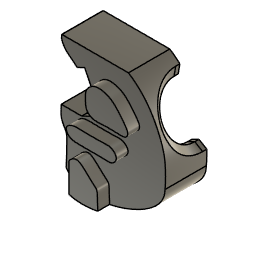
O4 Lite Cam Crux35 25° (Autodesk Fusion 360 design; units mm, degrees)
Autodesk Fusion 360 part; units mm, degrees
sketch "Skizze1" plane through (0, 0, 0) normal (0, 1, 0) x (1, 0, 0)
  spline S0 degree 5 poles (-4.5243, -6.4632) (-4.5158, -6.5005) (-4.4961, -6.5754) (-4.4576, -6.6893) (-4.387, -6.8464) (-4.2661, -7.0503) (-4.1148, -7.2567) (-3.9364, -7.4581) (-3.7332, -7.6461) (-3.5066, -7.8125) (-3.2573, -7.9501) (-2.9862, -8.0532) (-2.6953, -8.1181) (-2.3883, -8.144) (-2.0711, -8.1333) (-1.7509, -8.0908) (-1.4354, -8.0221) (-1.1309, -7.9326) (-0.8422, -7.8263) (-0.5706, -7.7044) (-0.3132, -7.5642) (-0.0646, -7.4007) (0.1819, -7.2085) (0.4324, -6.983) (0.6912, -6.7225) (0.9588, -6.4299) (1.2309, -6.1139) (1.4992, -5.7875) (1.7538, -5.4654) (1.9842, -5.1623) (2.1811, -4.8902) (2.3382, -4.6566) (2.4535, -4.4623) (2.5313, -4.2987) (2.5788, -4.1529) (2.6034, -4.0118) (2.6095, -3.8666) (2.5953, -3.7172) (2.5566, -3.5686) (2.4882, -3.4288) (2.3871, -3.3059) (2.253, -3.2064) (2.0873, -3.1347) (1.8932, -3.091) (1.6755, -3.0713) (1.4391, -3.0687) (1.1878, -3.0758) (0.9237, -3.0858) (0.6453, -3.0951) (0.3485, -3.1029) (0.0288, -3.1095) (-0.3168, -3.1156) (-0.6877, -3.1201) (-1.0785, -3.1204) (-1.4748, -3.1083) (-1.8652, -3.0861) (-2.2403, -3.0621) (-2.5925, -3.048) (-2.9161, -3.0556) (-3.2074, -3.0942) (-3.4642, -3.1674) (-3.6861, -3.2699) (-3.8741, -3.3904) (-4.0304, -3.5174) (-4.1583, -3.6426) (-4.2619, -3.7671) (-4.3457, -3.9025) (-4.4138, -4.0635) (-4.4694, -4.2624) (-4.5133, -4.5016) (-4.5449, -4.7733) (-4.5636, -5.0635) (-4.5705, -5.3549) (-4.5688, -5.6301) (-4.5684, -5.8739) (-4.5678, -6.0868) (-4.5607, -6.2401) (-4.5469, -6.3516) (-4.5327, -6.4259) (-4.5243, -6.4632) knots 0 0 0 0 0 0 0.01333333 0.02666667 0.04 0.05333333 0.06666667 0.08 0.09333333 0.10666667 0.12 0.13333333 0.14666667 0.16 0.17333333 0.18666667 0.2 0.21333333 0.22666667 0.24 0.25333333 0.26666667 0.28 0.29333333 0.30666667 0.32 0.33333333 0.34666667 0.36 0.37333333 0.38666667 0.4 0.41333333 0.42666667 0.44 0.45333333 0.46666667 0.48 0.49333333 0.50666667 0.52 0.53333333 0.54666667 0.56 0.57333333 0.58666667 0.6 0.61333333 0.62666667 0.64 0.65333333 0.66666667 0.68 0.69333333 0.70666667 0.72 0.73333333 0.74666667 0.76 0.77333333 0.78666667 0.8 0.81333333 0.82666667 0.84 0.85333333 0.86666667 0.88 0.89333333 0.90666667 0.92 0.93333333 0.94666667 0.96 0.97333333 0.98666667 1 1 1 1 1 1
  line L0 (-4.5692, -4.1589) -> (-4.5692, -6.8679)
  line L1 (0.5002, -3.1248) -> (-2.2874, -3.1136)
  spline S1 degree 5 poles (-7.828, 0.5821) (-7.8299, 0.5449) (-7.8288, 0.4718) (-7.8125, 0.3664) (-7.7619, 0.2361) (-7.6561, 0.0903) (-7.5159, -0.0401) (-7.3514, -0.156) (-7.1728, -0.2565) (-6.9877, -0.34) (-6.7987, -0.4054) (-6.6005, -0.4522) (-6.3797, -0.4819) (-6.1198, -0.4966) (-5.8052, -0.4996) (-5.4254, -0.4942) (-4.9796, -0.4843) (-4.4781, -0.4732) (-3.9383, -0.4641) (-3.3823, -0.4595) (-2.8342, -0.4609) (-2.3169, -0.4687) (-1.8502, -0.4819) (-1.4472, -0.4977) (-1.1118, -0.5117) (-0.8364, -0.517) (-0.6063, -0.5061) (-0.4046, -0.472) (-0.2155, -0.4094) (-0.03, -0.3161) (0.1518, -0.1938) (0.3238, -0.0463) (0.4756, 0.1215) (0.5947, 0.3046) (0.6695, 0.4998) (0.6907, 0.7037) (0.6542, 0.9119) (0.5635, 1.1178) (0.4316, 1.3115) (0.2757, 1.4821) (0.1115, 1.6204) (-0.0521, 1.7209) (-0.2189, 1.7847) (-0.4024, 1.8178) (-0.6194, 1.8292) (-0.8847, 1.8276) (-1.2051, 1.8201) (-1.5798, 1.811) (-2.0028, 1.8031) (-2.4635, 1.7979) (-2.9489, 1.7955) (-3.4452, 1.7953) (-3.9385, 1.7965) (-4.4173, 1.7979) (-4.8728, 1.7984) (-5.2979, 1.7967) (-5.6883, 1.7909) (-6.0413, 1.7786) (-6.3565, 1.7565) (-6.6355, 1.7204) (-6.8815, 1.6647) (-7.0991, 1.5836) (-7.2923, 1.4727) (-7.463, 1.3304) (-7.6098, 1.1597) (-7.7268, 0.9697) (-7.7902, 0.8116) (-7.8175, 0.695) (-7.8261, 0.6193) (-7.828, 0.5821) knots 0 0 0 0 0 0 0.01538462 0.03076923 0.04615385 0.06153846 0.07692308 0.09230769 0.10769231 0.12307692 0.13846154 0.15384615 0.16923077 0.18461538 0.2 0.21538462 0.23076923 0.24615385 0.26153846 0.27692308 0.29230769 0.30769231 0.32307692 0.33846154 0.35384615 0.36923077 0.38461538 0.4 0.41538462 0.43076923 0.44615385 0.46153846 0.47692308 0.49230769 0.50769231 0.52307692 0.53846154 0.55384615 0.56923077 0.58461538 0.6 0.61538462 0.63076923 0.64615385 0.66153846 0.67692308 0.69230769 0.70769231 0.72307692 0.73846154 0.75384615 0.76923077 0.78461538 0.8 0.81538462 0.83076923 0.84615385 0.86153846 0.87692308 0.89230769 0.90769231 0.92307692 0.93846154 0.95384615 0.96923077 0.98461538 1 1 1 1 1 1
  spline S2 degree 5 poles (0.7271, -10.9082) (0.7967, -10.8654) (0.9365, -10.7771) (1.1485, -10.6366) (1.4356, -10.4329) (1.8018, -10.1509) (2.1746, -9.8407) (2.553, -9.5012) (2.9346, -9.1301) (3.3165, -8.7247) (3.6952, -8.2828) (4.0668, -7.8031) (4.4273, -7.2869) (4.7731, -6.7381) (5.1012, -6.1651) (5.4088, -5.5784) (5.6938, -4.9891) (5.9542, -4.4067) (6.1884, -3.8372) (6.3948, -3.2812) (6.5719, -2.7314) (6.7184, -2.1753) (6.8338, -1.5992) (6.9185, -0.9921) (6.9744, -0.3496) (7.005, 0.3223) (7.0162, 1.0029) (7.0134, 1.663) (6.9995, 2.2713) (6.972, 2.8004) (6.9209, 3.2327) (6.8257, 3.5676) (6.6546, 3.8249) (6.3782, 4.033) (5.9781, 4.2204) (5.4612, 4.4038) (4.8576, 4.5875) (4.2094, 4.7688) (3.5631, 4.9413) (2.9601, 5.0993) (2.4284, 5.2416) (1.9725, 5.3758) (1.5805, 5.5149) (1.235, 5.6722) (0.9208, 5.8567) (0.6377, 6.0672) (0.4005, 6.2933) (0.2263, 6.5254) (0.1239, 6.7635) (0.0824, 7.0258) (0.0801, 7.3402) (0.0932, 7.7348) (0.1056, 8.2279) (0.1096, 8.8275) (0.1027, 9.5351) (0.0866, 10.3475) (0.0692, 11.0771) (0.0552, 11.6666) (0.0458, 12.0782) (0.041, 12.2887) knots 0 0 0 0 0 0 0.018182 0.036364 0.054545 0.072727 0.090909 0.109091 0.127273 0.145455 0.163636 0.181818 0.2 0.218182 0.236364 0.254545 0.272727 0.290909 0.309091 0.327273 0.345455 0.363636 0.381818 0.4 0.418182 0.436364 0.454545 0.472727 0.490909 0.509091 0.527273 0.545455 0.563636 0.581818 0.6 0.618182 0.636364 0.654545 0.672727 0.690909 0.709091 0.727273 0.745455 0.763636 0.781818 0.8 0.818182 0.836364 0.854545 0.872727 0.890909 0.909091 0.927273 0.945455 0.963636 0.981818 1 1 1 1 1 1
  line L2 (0.1295, 8.393) -> (-0.0476, 16.1843)
  spline S3 degree 5 poles (-10.5835, -10.8639) (-10.593, -10.8262) (-10.6087, -10.7498) (-10.6228, -10.632) (-10.6224, -10.4684) (-10.5903, -10.2535) (-10.5273, -10.0295) (-10.4348, -9.7988) (-10.3155, -9.5657) (-10.1726, -9.3361) (-10.0106, -9.1161) (-9.8339, -8.911) (-9.6472, -8.7244) (-9.4548, -8.5569) (-9.2607, -8.4053) (-9.0679, -8.2637) (-8.8786, -8.1254) (-8.6936, -7.9843) (-8.5125, -7.8363) (-8.3328, -7.6812) (-8.1517, -7.5217) (-7.9666, -7.3618) (-7.7768, -7.2058) (-7.5843, -7.057) (-7.3954, -6.9161) (-7.219, -6.7819) (-7.0644, -6.6516) (-6.9396, -6.5213) (-6.849, -6.3866) (-6.7922, -6.2435) (-6.7666, -6.0893) (-6.77, -5.9243) (-6.8027, -5.7531) (-6.8675, -5.5835) (-6.9667, -5.4229) (-7.1011, -5.2762) (-7.2676, -5.1432) (-7.4601, -5.0192) (-7.6714, -4.898) (-7.894, -4.7732) (-8.1219, -4.6398) (-8.3515, -4.4965) (-8.5808, -4.3444) (-8.8086, -4.1861) (-9.0343, -4.0251) (-9.2567, -3.865) (-9.4735, -3.7085) (-9.6808, -3.5567) (-9.8746, -3.4095) (-10.0503, -3.2646) (-10.2043, -3.1176) (-10.334, -2.9615) (-10.4384, -2.7872) (-10.518, -2.5853) (-10.5747, -2.3487) (-10.6116, -2.0738) (-10.6333, -1.7633) (-10.6449, -1.4252) (-10.6516, -1.0708) (-10.6581, -0.7128) (-10.6673, -0.3634) (-10.6804, -0.0325) (-10.6954, 0.2745) (-10.707, 0.5582) (-10.7075, 0.8239) (-10.6888, 1.0793) (-10.6445, 1.3319) (-10.5707, 1.5875) (-10.4688, 1.8472) (-10.3459, 2.1064) (-10.2126, 2.358) (-10.0811, 2.5943) (-9.9627, 2.8103) (-9.8663, 3.0054) (-9.7953, 3.1868) (-9.7489, 3.368) (-9.7229, 3.5636) (-9.7118, 3.7862) (-9.7104, 4.0413) (-9.7147, 4.3254) (-9.7214, 4.6299) (-9.7286, 4.9432) (-9.7349, 5.2537) (-9.7398, 5.5523) (-9.7434, 5.8358) (-9.7467, 6.1077) (-9.7506, 6.3758) (-9.7564, 6.65) (-9.7651, 6.9404) (-9.7773, 7.2548) (-9.7929, 7.5966) (-9.8113, 7.9641) (-9.8311, 8.3522) (-9.851, 8.7527) (-9.8693, 9.1564) (-9.8847, 9.5536) (-9.8961, 9.9353) (-9.9029, 10.2945) (-9.9054, 10.6272) (-9.9048, 10.9321) (-9.9035, 11.2096) (-9.9056, 11.4609) (-9.9168, 11.687) (-9.9451, 11.8882) (-10.0009, 12.0625) (-10.0906, 12.2077) (-10.2072, 12.3219) (-10.3222, 12.4063) (-10.3783, 12.4655) (-10.3182, 12.5059) (-10.1184, 12.5327) (-9.7918, 12.5498) (-9.3741, 12.5607) (-8.9151, 12.5693) (-8.4684, 12.5807) (-8.081, 12.6023) (-7.7844, 12.6437) (-7.5819, 12.7189) (-7.4552, 12.8428) (-7.3767, 13.0267) (-7.319, 13.2753) (-7.2672, 13.5814) (-7.2235, 13.9252) (-7.1974, 14.2804) (-7.1996, 14.6186) (-7.2347, 14.914) (-7.2939, 15.1483) (-7.3479, 15.3154) (-7.3413, 15.426) (-7.2152, 15.4984) (-6.9287, 15.5508) (-6.4787, 15.5938) (-5.8906, 15.6324) (-5.2103, 15.6666) (-4.4962, 15.6937) (-3.8111, 15.709) (-3.2139, 15.7075) (-2.7517, 15.6852) (-2.4513, 15.6403) (-2.312, 15.575) (-2.295, 15.4968) (-2.3237, 15.4181) (-2.3343, 15.3408) (-2.3181, 15.2438) (-2.295, 15.0995) (-2.2824, 14.8939) (-2.2806, 14.6331) (-2.2816, 14.3355) (-2.2708, 14.0265) (-2.2326, 13.7321) (-2.1539, 13.4735) (-2.0281, 13.2609) (-1.8548, 13.0959) (-1.6384, 12.9743) (-1.3877, 12.8884) (-1.1145, 12.8294) (-0.8332, 12.7902) (-0.5592, 12.7652) (-0.3075, 12.7499) (-0.0915, 12.7414) (0.0784, 12.7374) (0.1729, 12.7371) (0.2198, 12.7383) (0.2404, 12.7398) (0.248, 12.7407) knots 0 0 0 0 0 0 0.00625 0.0125 0.01875 0.025 0.03125 0.0375 0.04375 0.05 0.05625 0.0625 0.06875 0.075 0.08125 0.0875 0.09375 0.1 0.10625 0.1125 0.11875 0.125 0.13125 0.1375 0.14375 0.15 0.15625 0.1625 0.16875 0.175 0.18125 0.1875 0.19375 0.2 0.20625 0.2125 0.21875 0.225 0.23125 0.2375 0.24375 0.25 0.25625 0.2625 0.26875 0.275 0.28125 0.2875 0.29375 0.3 0.30625 0.3125 0.31875 0.325 0.33125 0.3375 0.34375 0.35 0.35625 0.3625 0.36875 0.375 0.38125 0.3875 0.39375 0.4 0.40625 0.4125 0.41875 0.425 0.43125 0.4375 0.44375 0.45 0.45625 0.4625 0.46875 0.475 0.48125 0.4875 0.49375 0.5 0.50625 0.5125 0.51875 0.525 0.53125 0.5375 0.54375 0.55 0.55625 0.5625 0.56875 0.575 0.58125 0.5875 0.59375 0.6 0.60625 0.6125 0.61875 0.625 0.63125 0.6375 0.64375 0.65 0.65625 0.6625 0.66875 0.675 0.68125 0.6875 0.69375 0.7 0.70625 0.7125 0.71875 0.725 0.73125 0.7375 0.74375 0.75 0.75625 0.7625 0.76875 0.775 0.78125 0.7875 0.79375 0.8 0.80625 0.8125 0.81875 0.825 0.83125 0.8375 0.84375 0.85 0.85625 0.8625 0.86875 0.875 0.88125 0.8875 0.89375 0.9 0.90625 0.9125 0.91875 0.925 0.93125 0.9375 0.94375 0.95 0.95625 0.9625 0.96875 0.975 0.98125 0.9875 0.99375 1 1 1 1 1 1
  spline S4 degree 5 poles (-10.5835, -10.8639) (-10.58, -10.8789) (-10.5697, -10.9076) (-10.5442, -10.9472) (-10.4901, -10.9926) (-10.3892, -11.0376) (-10.2564, -11.0718) (-10.0953, -11.0974) (-9.9126, -11.1185) (-9.7173, -11.1407) (-9.5195, -11.17) (-9.3291, -11.212) (-9.1547, -11.2716) (-9.0019, -11.3517) (-8.8735, -11.4531) (-8.7699, -11.5755) (-8.6903, -11.7173) (-8.6331, -11.877) (-8.5967, -12.053) (-8.5799, -12.244) (-8.5817, -12.4493) (-8.5976, -12.6245) (-8.6174, -12.762) (-8.6341, -12.8563) (-8.6433, -12.9041) knots 0 0 0 0 0 0 0.05 0.1 0.15 0.2 0.25 0.3 0.35 0.4 0.45 0.5 0.55 0.6 0.65 0.7 0.75 0.8 0.85 0.9 0.95 1 1 1 1 1 1
  line L3 (-8.6433, -12.9041) -> (1.0723, -12.9041)
  line L4 (0.7271, -10.9082) -> (0.7271, -12.9041)
  line L5 (0.041, 12.2887) -> (0.0307, 12.7389)
  spline S5 degree 5 poles (-7.3471, 5.0204) (-7.3368, 5.0013) (-7.3139, 4.9624) (-7.2723, 4.9023) (-7.2022, 4.819) (-7.0909, 4.7099) (-6.9574, 4.5983) (-6.8045, 4.4885) (-6.637, 4.388) (-6.4609, 4.3055) (-6.282, 4.249) (-6.1051, 4.2247) (-5.9336, 4.2347) (-5.768, 4.2765) (-5.6073, 4.3456) (-5.4491, 4.4366) (-5.29, 4.5454) (-5.1262, 4.6706) (-4.9538, 4.8134) (-4.7697, 4.9751) (-4.5719, 5.1566) (-4.3602, 5.3568) (-4.137, 5.5713) (-3.9072, 5.7915) (-3.6777, 6.0072) (-3.4561, 6.2083) (-3.25, 6.3867) (-3.0664, 6.5386) (-2.9105, 6.6658) (-2.7847, 6.7787) (-2.6891, 6.8941) (-2.6212, 7.0302) (-2.5773, 7.2024) (-2.5523, 7.418) (-2.5403, 7.674) (-2.5355, 7.9606) (-2.5327, 8.2638) (-2.5275, 8.5679) (-2.5177, 8.8589) (-2.503, 9.1266) (-2.4863, 9.3678) (-2.4724, 9.5842) (-2.467, 9.7804) (-2.4758, 9.9615) (-2.5031, 10.1314) (-2.5511, 10.2904) (-2.62, 10.4356) (-2.709, 10.5628) (-2.8174, 10.6681) (-2.9453, 10.7498) (-3.0942, 10.8089) (-3.2659, 10.8481) (-3.4616, 10.8716) (-3.6814, 10.8837) (-3.9234, 10.8886) (-4.1844, 10.8905) (-4.46, 10.8924) (-4.7449, 10.8966) (-5.0331, 10.904) (-5.3186, 10.9142) (-5.5952, 10.9248) (-5.8572, 10.932) (-6.0998, 10.9319) (-6.3192, 10.9202) (-6.5131, 10.8935) (-6.6812, 10.8495) (-6.8254, 10.7879) (-6.9487, 10.7091) (-7.0547, 10.6145) (-7.1464, 10.5053) (-7.2256, 10.3823) (-7.2798, 10.2731) (-7.3154, 10.1853) (-7.3369, 10.124) (-7.3471, 10.0927) knots 0 0 0 0 0 0 0.01428571 0.02857143 0.04285714 0.05714286 0.07142857 0.08571429 0.1 0.11428571 0.12857143 0.14285714 0.15714286 0.17142857 0.18571429 0.2 0.21428571 0.22857143 0.24285714 0.25714286 0.27142857 0.28571429 0.3 0.31428571 0.32857143 0.34285714 0.35714286 0.37142857 0.38571429 0.4 0.41428571 0.42857143 0.44285714 0.45714286 0.47142857 0.48571429 0.5 0.51428571 0.52857143 0.54285714 0.55714286 0.57142857 0.58571429 0.6 0.61428571 0.62857143 0.64285714 0.65714286 0.67142857 0.68571429 0.7 0.71428571 0.72857143 0.74285714 0.75714286 0.77142857 0.78571429 0.8 0.81428571 0.82857143 0.84285714 0.85714286 0.87142857 0.88571429 0.9 0.91428571 0.92857143 0.94285714 0.95714286 0.97142857 0.98571429 1 1 1 1 1 1
  line L6 (-7.3471, 5.0204) -> (-7.3471, 10.0927)
  line L7 (0.7271, -10.9082) -> (-10.5662, -10.9082)
  spline S6 degree 5 poles (1.0592, 5.7812) (0.6047, 5.9716) (-0.3091, 6.3124) (-1.6948, 6.7027) (-3.5583, 6.9827) (-5.8366, 6.8357) (-7.5331, 6.1361) (-8.682, 5.1382) (-9.3829, 4.2305) (-9.717, 3.7159) knots 0 0 0 0 0 0 0.2 0.4 0.6 0.8 1 1 1 1 1 1
  line L8 (2.1287, 5.3329) -> (-0.0104, 6.2295)
  line L9 (-8.9784, 4.8533) -> (-10.4557, 2.5786)
  spline S7 degree 5 poles (6.9248, 3.125) (6.9282, 3.4844) (6.8431, 4.1897) (6.4398, 5.2074) (5.3882, 6.4762) (3.4261, 7.8713) (1.0807, 9.0146) (-1.3779, 9.8419) (-3.7125, 10.2975) (-5.773, 10.3603) (-7.4988, 10.0428) (-8.5998, 9.5018) (-9.2721, 8.9435) (-9.6531, 8.5047) (-9.8268, 8.2686) knots 0 0 0 0 0 0 0.1 0.2 0.3 0.4 0.5 0.6 0.7 0.8 0.9 1 1 1 1 1 1
  line L10 (6.911, 1.683) -> (6.9386, 4.5671)
  point P0 (-4.0016, -7.3793)
  point P1 (-2.6808, -8.1099)
  point P2 (-0.8486, -7.8233)
  point P3 (0.7025, -6.7049)
  point P4 (2.3324, -4.6591)
  point P5 (2.5965, -4.0297)
  point P6 (2.5347, -3.5351)
  point P7 (2.1132, -3.1529)
  point P8 (1.0847, -3.0799)
  point P9 (-0.8936, -3.1192)
  point P10 (-3.2485, -3.1136)
  point P11 (-4.114, -3.6025)
  point P12 (-4.4343, -4.1477)
  point P13 (-4.5692, -5.5134)
  point P14 (-7.563, 0.0092)
  point P15 (-6.8669, -0.379)
  point P16 (-5.6039, -0.496)
  point P17 (-1.4945, -0.496)
  point P18 (-0.2685, -0.4221)
  point P19 (0.4585, 0.1139)
  point P20 (0.6434, 0.9025)
  point P21 (0.0766, 1.6356)
  point P22 (-0.6689, 1.8266)
  point P23 (-3.5954, 1.7958)
  point P24 (-6.4602, 1.7404)
  point P25 (-7.4398, 1.3399)
  point P26 (2.3872, -9.6465)
  point P27 (4.4678, -7.2117)
  point P28 (6.2386, -3.6923)
  point P29 (6.969, -0.3279)
  point P30 (6.9248, 3.125)
  point P31 (6.2165, 4.099)
  point P32 (2.8963, 5.1171)
  point P33 (1.0592, 5.7812)
  point P34 (0.2402, 6.5337)
  point P35 (0.0852, 7.4412)
  point P36 (-10.4741, -9.9052)
  point P37 (-9.6406, -8.7243)
  point P38 (-8.6751, -7.9672)
  point P39 (-7.7444, -7.1823)
  point P40 (-6.9734, -6.5502)
  point P41 (-6.7719, -6.0432)
  point P42 (-6.9873, -5.4111)
  point P43 (-7.8694, -4.786)
  point P44 (-9.1544, -3.9385)
  point P45 (-10.1546, -3.1606)
  point P46 (-10.5835, -2.2576)
  point P47 (-10.6825, -0.0002)
  point P48 (-10.5835, 1.528)
  point P49 (-9.9324, 2.8755)
  point P50 (-9.717, 3.7159)
  point P51 (-9.7379, 5.4455)
  point P52 (-9.7719, 7.1063)
  point P53 (-9.8968, 10.0068)
  point P54 (-9.9245, 11.7137)
  point P55 (-10.2021, 12.3105)
  point P56 (-10.3409, 12.477)
  point P57 (-8.0233, 12.6158)
  point P58 (-7.3432, 13.1848)
  point P59 (-7.2877, 15.1138)
  point P60 (-7.1906, 15.4885)
  point P61 (-2.3611, 15.5857)
  point P62 (-2.3194, 15.4191)
  point P63 (-2.3056, 15.1555)
  point P64 (-2.2223, 13.7399)
  point P65 (-1.3758, 12.8934)
  point P66 (-0.0435, 12.7407)
  point P67 (-10.2162, -11.0761)
  point P68 (-9.2385, -11.2462)
  point P69 (-8.6646, -11.7988)
  point P70 (-6.9606, 4.605)
  point P71 (-6.1684, 4.2379)
  point P72 (-5.4341, 4.4504)
  point P73 (-4.41, 5.3103)
  point P74 (-3.0091, 6.5856)
  point P75 (-2.5936, 7.1556)
  point P76 (-2.5164, 8.8561)
  point P77 (-2.4874, 10.0154)
  point P78 (-2.7676, 10.6144)
  point P79 (-3.4342, 10.8656)
  point P80 (-5.0187, 10.9043)
  point P81 (-6.4776, 10.8946)
  point P82 (-7.0476, 10.6144)
  point P83 (-2.4874, 10.0154)
  constraint midpoint P13 L0
  constraint midpoint P9 L1
  constraint midpoint S2.end L2
  constraint horizontal L3
  constraint coincident L3 L4.end
  constraint perpendicular L3 L4
  constraint coincident S3 L5.end
  constraint vertical L6
  constraint horizontal L7
  constraint coincident S4 L7.end
  constraint coincident P33 S6.start
  constraint coincident P50 S6.end
  constraint midpoint P33 L8
  constraint coincident S2 L8.start
  constraint midpoint P50 L9
  constraint coincident P30 S7.start
  constraint coincident P83 P77
  constraint midpoint P30 L10
  constraint coincident S3 S7.end
extrude "Extrusion1" add sketch "Skizze1" along normal blind 1 contours S0 | S1 | S2 S3 S4 S5 L6 L7 S6 | S2 L2 S7 | S4 L3 L4 L7 | S2 S5 S6 S7 | S2 L2 S3 L5 S5 L6 S7 | S3 L6 S6 S7 | S5 L6 S6 S7 | S5 L6 S6 | S5 L6 S7 makes body 1
extrude "Extrusion2" add sketch "Skizze1" along normal blind 3 contours S0 | S1 | S5 L6 S6 S7 | S5 L6 S6 | S5 L6 S7 bodies 1
delete_body "Körper entfernen1" bodies 1
sketch "Skizze2" plane through (0, 0, 0) normal (1, 0, 0) x (0, 1, 0)
  line L0 (0, 0) -> (14, 0)
  circle A0 centre (7, 0) radius 4.3
  line L1 (12.5, -5.5) -> (1.5, -5.5)
  line L2 (1.5, -5.5) -> (1.5, 5.5)
  line L3 (1.5, 5.5) -> (12.5, 5.5)
  line L4 (12.5, 5.5) -> (12.5, -5.5)
  line L5 (12.5, -5.5) -> (1.5, 5.5) construction
  line L6 (1.5, -5.5) -> (12.5, 5.5) construction
  line L7 (13.1, -6.1) -> (0.9, -6.1)
  line L8 (0.9, -6.1) -> (0.9, 6.1)
  line L9 (0.9, 6.1) -> (13.1, 6.1)
  line L10 (13.1, 6.1) -> (13.1, -6.1)
  line L11 (13.1, -6.1) -> (0.9, 6.1) construction
  line L12 (0.9, -6.1) -> (13.1, 6.1) construction
  line L13 (13.25, -8.25) -> (0.75, -8.25)
  line L14 (0.75, -8.25) -> (0.75, 8.25)
  line L15 (0.75, 8.25) -> (13.25, 8.25)
  line L16 (13.25, 8.25) -> (13.25, -8.25)
  line L17 (13.25, -8.25) -> (0.75, 8.25) construction
  line L18 (0.75, -8.25) -> (13.25, 8.25) construction
  point P0 (7, 0)
  point P1 (7, 0)
  point P2 (7, 0)
  dimension "d5" = 14
  dimension "d6" = 8.6
  dimension "d7" = 11
  dimension "d8" = 11
  dimension "d9" = 12.2
  dimension "d10" = 12.2
  dimension "d11" = 12.5
  dimension "d12" = 16.5
  constraint coincident L0.start origin
  constraint horizontal L0
  constraint midpoint L0 P2
  constraint horizontal L1
  constraint perpendicular L1 L2
  constraint parallel L1 L3
  constraint parallel L2 L4
  constraint coincident L5 P2
  constraint coincident L6 P2
  constraint coincident P2 P1
  constraint horizontal L7
  constraint perpendicular L7 L8
  constraint parallel L7 L9
  constraint parallel L8 L10
  constraint coincident L11 P2
  constraint coincident L12 P2
  constraint horizontal L13
  constraint perpendicular L13 L14
  constraint parallel L13 L15
  constraint parallel L14 L16
  constraint coincident L17 P2
  constraint coincident L18 P2
  measures "d5" distance of L0.start L0.end
  measures "d6" diameter of A0
  measures "d7" distance of L2.end L3.end
  measures "d8" distance of L1.end L2.end
  measures "d9" distance of L8.end L9.end
  measures "d10" distance of L7.end L8.end
  measures "d11" distance of L14.end L15.end
  measures "d12" distance of L13.end L14.end
extrude "Extrusion3" add sketch "Skizze1" along normal blind 7 separate body contours S0 | S1 | S2 S3 S4 S5 L6 L7 S6 | S5 L6 S6 makes body 2
sketch "Skizze3" plane through (0, 7, 0) normal (0, 1, 0) x (-1, 0, 0)
  spline S0 degree 5 poles (-0.7271, 10.9082) (-0.7967, 10.8654) (-0.9365, 10.7771) (-1.1485, 10.6366) (-1.4356, 10.4329) (-1.8018, 10.1509) (-2.1746, 9.8407) (-2.553, 9.5012) (-2.9346, 9.1301) (-3.3165, 8.7247) (-3.6952, 8.2828) (-4.0668, 7.8031) (-4.4273, 7.2869) (-4.7731, 6.7381) (-5.1012, 6.1651) (-5.4088, 5.5784) (-5.6938, 4.9891) (-5.9542, 4.4067) (-6.1884, 3.8372) (-6.3948, 3.2812) (-6.5719, 2.7314) (-6.7184, 2.1753) (-6.8338, 1.5992) (-6.9185, 0.9921) (-6.9744, 0.3496) (-7.005, -0.3223) (-7.0162, -1.0029) (-7.0134, -1.663) (-6.9995, -2.2713) (-6.972, -2.8004) (-6.9209, -3.2327) (-6.8257, -3.5676) (-6.6546, -3.8249) (-6.3782, -4.033) (-5.9781, -4.2204) (-5.4612, -4.4038) (-4.8576, -4.5875) (-4.2094, -4.7688) (-3.5631, -4.9413) (-2.9601, -5.0993) (-2.4284, -5.2416) (-1.9725, -5.3758) (-1.6141, -5.503) (-1.3636, -5.614) (-1.1944, -5.7025) (-1.0949, -5.7599) (-1.0592, -5.7812) knots 0 0 0 0 0 0 0.018182 0.036364 0.054545 0.072727 0.090909 0.109091 0.127273 0.145455 0.163636 0.181818 0.2 0.218182 0.236364 0.254545 0.272727 0.290909 0.309091 0.327273 0.345455 0.363636 0.381818 0.4 0.418182 0.436364 0.454545 0.472727 0.490909 0.509091 0.527273 0.545455 0.563636 0.581818 0.6 0.618182 0.636364 0.654545 0.672727 0.690909 0.709091 0.727273 0.745455 0.75586 0.75586 0.75586 0.75586 0.75586 0.75586
  spline S1 degree 5 poles (-1.0592, -5.7812) (-0.6047, -5.9716) (0.3091, -6.3124) (1.6948, -6.7027) (3.5583, -6.9827) (5.8366, -6.8357) (7.5331, -6.1361) (8.682, -5.1382) (9.3829, -4.2305) (9.717, -3.7159) knots 0 0 0 0 0 0 0.2 0.4 0.6 0.8 1 1 1 1 1 1
  spline S2 degree 5 poles (9.717, -3.7159) (9.7184, -3.6855) (9.7224, -3.6111) (9.7317, -3.4983) (9.752, -3.3558) (9.7953, -3.1868) (9.8663, -3.0054) (9.9627, -2.8103) (10.0811, -2.5943) (10.2126, -2.358) (10.3459, -2.1064) (10.4688, -1.8472) (10.5707, -1.5875) (10.6445, -1.3319) (10.6888, -1.0793) (10.7075, -0.8239) (10.707, -0.5582) (10.6954, -0.2745) (10.6804, 0.0325) (10.6673, 0.3634) (10.6581, 0.7128) (10.6516, 1.0708) (10.6449, 1.4252) (10.6333, 1.7633) (10.6116, 2.0738) (10.5747, 2.3487) (10.518, 2.5853) (10.4384, 2.7872) (10.334, 2.9615) (10.2043, 3.1176) (10.0503, 3.2646) (9.8746, 3.4095) (9.6808, 3.5567) (9.4735, 3.7085) (9.2567, 3.865) (9.0343, 4.0251) (8.8086, 4.1861) (8.5808, 4.3444) (8.3515, 4.4965) (8.1219, 4.6398) (7.894, 4.7732) (7.6714, 4.898) (7.4601, 5.0192) (7.2676, 5.1432) (7.1011, 5.2762) (6.9667, 5.4229) (6.8675, 5.5835) (6.8027, 5.7531) (6.77, 5.9243) (6.7666, 6.0893) (6.7922, 6.2435) (6.849, 6.3866) (6.9396, 6.5213) (7.0644, 6.6516) (7.219, 6.7819) (7.3954, 6.9161) (7.5843, 7.057) (7.7768, 7.2058) (7.9666, 7.3618) (8.1517, 7.5217) (8.3328, 7.6812) (8.5125, 7.8363) (8.6936, 7.9843) (8.8786, 8.1254) (9.0679, 8.2637) (9.2607, 8.4053) (9.4548, 8.5569) (9.6472, 8.7244) (9.8339, 8.911) (10.0106, 9.1161) (10.1726, 9.3361) (10.3155, 9.5657) (10.4348, 9.7988) (10.5273, 10.0295) (10.5903, 10.2535) (10.6224, 10.4684) (10.6228, 10.632) (10.6087, 10.7498) (10.593, 10.8262) (10.5835, 10.8639) knots -0.46665611 -0.46665611 -0.46665611 -0.46665611 -0.46665611 -0.46665611 -0.4625 -0.45625 -0.45 -0.44375 -0.4375 -0.43125 -0.425 -0.41875 -0.4125 -0.40625 -0.4 -0.39375 -0.3875 -0.38125 -0.375 -0.36875 -0.3625 -0.35625 -0.35 -0.34375 -0.3375 -0.33125 -0.325 -0.31875 -0.3125 -0.30625 -0.3 -0.29375 -0.2875 -0.28125 -0.275 -0.26875 -0.2625 -0.25625 -0.25 -0.24375 -0.2375 -0.23125 -0.225 -0.21875 -0.2125 -0.20625 -0.2 -0.19375 -0.1875 -0.18125 -0.175 -0.16875 -0.1625 -0.15625 -0.15 -0.14375 -0.1375 -0.13125 -0.125 -0.11875 -0.1125 -0.10625 -0.1 -0.09375 -0.0875 -0.08125 -0.075 -0.06875 -0.0625 -0.05625 -0.05 -0.04375 -0.0375 -0.03125 -0.025 -0.01875 -0.0125 -0.00625 0 0 0 0 0 0
  spline S3 degree 5 poles (10.5835, 10.8639) (10.5813, 10.8732) (10.5785, 10.8823) (10.5751, 10.8911) (10.5709, 10.8998) (10.5662, 10.9082) knots 0 0 0 0 0 0 0.031102 0.031102 0.031102 0.031102 0.031102 0.031102
  line L0 (10.5662, 10.9082) -> (-0.7271, 10.9082)
  line L1 (-0.7271, 10.9082) -> (-1.0592, -5.7812) construction
  line L2 (-0.8931, 2.5635) -> (-7.1772, 5.6474) construction
  line L3 (-5.7158, 4.9302) -> (-2.5737, 3.3883)
  line L4 (-2.5737, 3.3883) -> (-0.1507, 8.3257)
  line L5 (-0.1507, 8.3257) -> (4.1584, 6.211)
  line L6 (4.1584, 6.211) -> (4.4227, 6.7497)
  line L7 (-0.1507, 8.3257) -> (1.3978, 11.481)
  line L8 (4.4227, 6.7497) -> (0.1137, 8.8644)
  line L9 (0.1137, 8.8644) -> (5.7693, 6.0888)
  line L10 (-2.5737, 3.3883) -> (1.0389, 10.7496)
  line L11 (1.0389, 10.7496) -> (7.9561, 7.3549)
  line L12 (5.7693, 6.0888) -> (6.6945, 7.974)
  line L13 (-0.8931, 2.5635) -> (7.0521, -1.3357) construction
  line L14 (4.1584, 6.211) -> (1.7353, 1.2736)
  line L15 (5.7693, 6.0888) -> (3.0819, 0.6127)
  line L16 (-2.5737, 3.3883) -> (-4.9968, -1.5492)
  line L17 (-4.9968, -1.5492) -> (-0.6878, -3.6639)
  line L18 (-0.6878, -3.6639) -> (1.7353, 1.2736)
  line L19 (-0.6878, -3.6639) -> (-0.9521, -4.2025)
  line L20 (-5.2612, -2.0879) -> (0.3945, -4.8634)
  line L21 (0.3945, -4.8634) -> (3.0819, 0.6127)
  line L22 (0.3945, -4.8634) -> (-0.5307, -6.7486)
  line L23 (-6.1863, -3.9731) -> (2.7909, -8.3787)
  line L24 (-6.1863, -3.9731) -> (2.7909, -8.3787)
  line L25 (2.7909, -8.3787) -> (7.1965, 0.5985)
  line L26 (7.1965, 0.5985) -> (11.7126, 0.5985)
  line L27 (7.1965, 0.5985) -> (3.8749, 2.2286)
  line L28 (7.9561, 7.3549) -> (11.7126, 7.3549)
  line L29 (11.7126, 7.3549) -> (11.7126, 0.5985)
  dimension "d16" = 65
  dimension "d17" = 7
  dimension "d18" = 3.5
  dimension "d19" = 5.5
  dimension "d21" = 4.8
  dimension "d22" = 0.6
  dimension "d23" = 6.3
  dimension "d24" = 8.2
  dimension "d27" = 10
  dimension "d28" = 10
  constraint coincident S0.start L0.end
  constraint coincident S0.end S1.start
  constraint midpoint L1 L2.start
  constraint coincident S0 L3.start
  constraint coincident L2 L3.start
  constraint parallel L2 L3
  constraint perpendicular L3 L4
  constraint perpendicular L4 L5
  constraint perpendicular L5 L6
  constraint perpendicular L5 L7
  constraint coincident L7 L8.end
  constraint perpendicular L7 L8
  constraint perpendicular L6 L9
  constraint perpendicular L3 L10
  constraint perpendicular L7 L11
  constraint coincident L11 L12.end
  constraint perpendicular L11 L12
  constraint parallel L2 L13
  constraint coincident L13 L14.end
  constraint perpendicular L13 L14
  constraint coincident L13 L15.end
  constraint perpendicular L13 L15
  constraint symmetric L2 L3.end L4.start
  constraint symmetric L2 L4.end L16.end
  constraint symmetric L2 L5.end L17.end
  constraint symmetric L2 L6.end L19.end
  constraint symmetric L2 L8.end L20.start
  constraint symmetric L2 L9.end L20.end
  constraint symmetric L2 L10.end L23.start
  constraint symmetric L2 L12.end L22.end
  constraint symmetric L2 L14.end L18.end
  constraint symmetric L2 L15.end L21.end
  constraint parallel L23 L24
  constraint perpendicular L24 L25
  constraint horizontal L26
  constraint coincident L15 L27.end
  constraint perpendicular L15 L27
  constraint coincident S2 L11.end
  constraint parallel L26 L28
  constraint perpendicular L26 L29
  measures "d16" angle of L1 L2
  measures "d17" distance of L2.start L2.end
  measures "d18" distance of L3.start L3.end
  measures "d19" distance of L3.end L4.end
  measures "d21" distance of L4.end L5.end
  measures "d22" distance of L5.end L6.end
  measures "d23" distance of L8.end L9.end
  measures "d24" distance of L3.end L10.end
  measures "d27" distance of L23.start L23.end
  measures "d28" distance of L23.end L25.end
extrude "Extrusion4" add sketch "Skizze1" along normal blind 7 contours S2 L8 S7 | S2 L8 | S2 S5 S6 S7 | S3 L6 S6 S7 | S5 L6 S6 S7 bodies 2
extrude "Extrusion5" cut sketch "Skizze3" against normal blind 5.5 contours L4 L5 L10 L14 L16 L17 L18 bodies 2
extrude "Extrusion6" cut sketch "Skizze3" against normal blind 6.1 contours L6 L9 L14 L15 L18 L19 L20 L21 bodies 2
extrude "Extrusion7" cut sketch "Skizze3" against normal blind 6.25 contours S1 L22 L23 L24 L25 | S1 L15 L21 L22 L25 L27 bodies 2
extrude "Extrusion8" cut sketch "Skizze3" against normal blind 7 contours S2 L11 L12 L15 L26 L27 bodies 2
extrude "Extrusion9" add sketch "Skizze1" against normal blind 2 contours S0 | S1 | S5 L6 S6 S7 | S5 L6 S6 bodies 2
sketch "Skizze5" plane through (3.4143, 0, 1.6756) normal (-0.897723, 0, -0.440561) x (0, -1, 0)
  line L0 (-7, 7.4078) -> (-7, -3.5922)
  line L1 (-7, -3.5922) -> (-1.5, -3.5922)
  line L2 (-1.5, -3.5922) -> (-1.5, 7.4078)
  line L3 (-1.5, 7.4078) -> (-7, 7.4078)
  line L4 (-7, 1.9078) -> (-6.3, 1.9078)
  line L5 (-6.3, 6.2078) -> (-7, 6.2078)
  line L6 (-6.3, 1.9078) -> (-6.3, -2.3922) construction
  line L7 (-7, 6.2078) -> (-7, -3.0088)
  line L8 (-6.3, -2.3922) -> (-7, -2.3922)
  arc A0 (-6.3, -2.3922) -> (-6.3, 6.2078) centre (-6.3, 1.9078) ccw
  dimension "d45" = 0.7
  dimension "d46" = 8.6
  constraint midpoint L0 L4.start
  constraint perpendicular L0 L4
  constraint coincident L4.end L6.start
  constraint coincident L0 L5.end
  constraint tangent L5 A0
  constraint perpendicular L4 L6
  constraint coincident L0 L7.end
  constraint perpendicular L5 L7
  constraint horizontal L8
  constraint coincident L7 L8.end
  measures "d45" distance of L4.start L4.end
  measures "d46" diameter of A0
extrude "Extrusion11" cut sketch "Skizze5" against normal blind 11 bodies 2
extrude "Extrusion12" add sketch "Skizze3" against normal blind 5.5 contours S0 L0 L3 L4 L7 L10 | S0 S1 L3 L16 L17 L19 L20 L22 bodies 2
extrude "Extrusion13" cut sketch "Skizze5" against normal blind 15 contours L0 L5 L7 L8 A0 bodies 2
chamfer "Fase2" distance 1.4 angle 45 3 edges at (5.721, 2, 4.9189) (3.4226, 6.65, 8.5948) (6.9365, 6.65, 0.7394) on bodies 2
extrude "Extrusion10" [suppressed]
equation "d16 = 90 deg - 25 deg"
equation "d24 = ( 16.4 / 2 ) * 1 mm"
equation "d31 = ( -12.2 / 2 ) * 1 mm"
equation "d33 = ( -12.5 / 2 ) * 1 mm"
